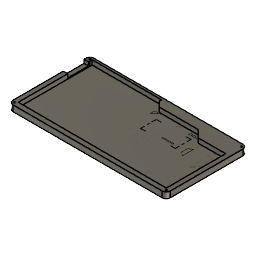
bottom (Autodesk Fusion 360 design; units mm, degrees)
part number: 2026-05-11-22-57-26-323
Autodesk Fusion 360 part; units mm, degrees
sketch "Sketch2" plane through (0, 0, 0) normal (0, 0, 1) x (1, 0, 0)
  line L0 (-104.034, 27.8554) -> (-104.2569, -127.6847)
  line L1 (47.3447, 27.8244) -> (-104.034, 27.8554)
  line L2 (58.096, 16.7354) -> (47.3447, 27.8244)
  line L3 (143.396, 16.6254) -> (58.096, 16.7354)
  line L4 (158.776, 0.9754) -> (143.396, 16.6254)
  line L5 (218.636, 1.1054) -> (158.776, 0.9754)
  line L6 (218.786, -128.4147) -> (218.636, 1.1054)
  line L7 (-104.2569, -127.6847) -> (218.786, -128.4147)
  line L8 (-114.034, 37.8554) -> (228.636, 37.8554)
  line L9 (228.636, 37.8554) -> (228.636, -138.4147)
  line L10 (228.636, -138.4147) -> (-114.034, -138.4147)
  line L11 (-114.034, -138.4147) -> (-114.034, 37.8554)
  circle A0 centre (-108.034, 31.8554) radius 1.75
  circle A1 centre (222.636, 31.8554) radius 1.75
  circle A2 centre (-108.034, -132.4147) radius 1.75
  circle A3 centre (222.636, -132.4147) radius 1.75
  dimension "d24" = 10
  dimension "d25" = 10
  dimension "d26" = 10
  dimension "d27" = 10
  dimension "d32" = 3.5
  dimension "d33" = 6
  dimension "d34" = 6
  dimension "d35" = 6
  dimension "d36" = 6
  dimension "d37" = 3.5
  dimension "d38" = 3.5
  dimension "d39" = 6
  dimension "d40" = 6
  dimension "d41" = 3.5
  dimension "d42" = 6
  dimension "d43" = 6
  constraint horizontal L8
  constraint vertical L9
  constraint horizontal L10
  constraint vertical L11
  measures "d24" vertical distance of L0.start L8.start
  measures "d25" distance of L0.start L11
  measures "d26" horizontal distance of L5.start L8.end
  measures "d27" vertical distance of L6.start L9.end
  measures "d32" diameter of A0
  measures "d33" distance of L8 A0.centre
  measures "d34" distance of L11 A0.centre
  measures "d35" distance of L9 A1.centre
  measures "d36" distance of L8 A1.centre
  measures "d37" diameter of A1
  measures "d38" diameter of A2
  measures "d39" distance of L11 A2.centre
  measures "d40" distance of L10 A2.centre
  measures "d41" diameter of A3
  measures "d42" distance of L9 A3.centre
  measures "d43" distance of L10 A3.centre
extrude "Extrude2" add sketch "Sketch2" along normal blind 3 contours L0 L1 L2 L3 L4 L5 L6 L7
extrude "Extrude3" add sketch "Sketch2" along normal blind 13 contours L8 L9 L10 L11 | A0 | A1 | A2 | A3
sketch "Sketch5" plane through (0, 0, 13) normal (0, 0, 1) x (-1, 0, 0)
  line L0 (-218.786, 128.4147) -> (104.2569, 127.6847)
  line L1 (104.2569, 127.6847) -> (104.034, -27.8554)
  line L2 (104.034, -27.8554) -> (-47.3447, -27.8244)
  line L3 (-47.3447, -27.8244) -> (-58.096, -16.7354)
  line L4 (-58.096, -16.7354) -> (-143.396, -16.6254)
  line L5 (-143.396, -16.6254) -> (-158.776, -0.9754)
  line L6 (-158.776, -0.9754) -> (-218.636, -1.1054)
  line L7 (-218.636, -1.1054) -> (-218.786, 128.4147)
  line L8 (114.034, 138.4147) -> (-228.636, 138.4147)
  line L9 (-228.636, 138.4147) -> (-228.636, -37.8554)
  line L10 (-228.636, -37.8554) -> (114.034, -37.8554)
  line L11 (114.034, -37.8554) -> (114.034, 138.4147)
  circle A0 centre (108.034, -31.8554) radius 1.75
  line L12 (114.034, -37.8554) -> (-228.636, -37.8554)
  line L13 (114.034, 138.4147) -> (114.034, -37.8554)
  circle A1 centre (108.034, 132.4147) radius 1.75
  line L14 (-228.636, 138.4147) -> (114.034, 138.4147)
  circle A2 centre (-222.636, 132.4147) radius 1.75
  line L15 (-228.636, -37.8554) -> (-228.636, 138.4147)
  circle A3 centre (-222.636, -31.8554) radius 1.75
  dimension "d44" = 3.5
  dimension "d45" = 6
  dimension "d46" = 6
  dimension "d47" = 3.5
  dimension "d48" = 6
  dimension "d49" = 6
  dimension "d50" = 3.5
  dimension "d51" = 6
  dimension "d52" = 6
  dimension "d53" = 3.5
  dimension "d54" = 6
  dimension "d55" = 6
  measures "d44" diameter of A0
  measures "d45" distance of A0.centre L12
  measures "d46" distance of A0.centre L13
  measures "d47" diameter of A1
  measures "d48" distance of A1.centre L14
  measures "d49" distance of L13 A1.centre
  measures "d50" diameter of A2
  measures "d51" distance of A2.centre L15
  measures "d52" distance of L14 A2.centre
  measures "d53" diameter of A3
  measures "d54" distance of L15 A3.centre
  measures "d55" distance of L12 A3.centre
extrude "Extrude4" cut sketch "Sketch5" against normal blind 13 contours A0 | A1 | A2 | A3
fillet "Fillet1" radius 9 4 edges at (-114.034, -138.4147, 6.5) (228.636, -138.4147, 6.5) (228.636, 37.8554, 6.5) (-114.034, 37.8554, 6.5)
sketch "Sketch6" plane through (-114.034, 0, 0) normal (-1, 0, 0) x (0, -1, 0)
  line L0 (-28.8554, 13) -> (-28.8554, 0)
  line L1 (-28.8554, 0) -> (129.4147, 0)
  line L2 (129.4147, 0) -> (129.4147, 13)
  line L3 (129.4147, 13) -> (-28.8554, 13)
  line L4 (-25.142, 13) -> (20, 13)
  line L5 (20, 13) -> (20, 5)
  line L6 (20, 5) -> (-25.142, 5)
  line L7 (-25.142, 5) -> (-25.142, 13)
  constraint horizontal L4
  constraint vertical L5
  constraint horizontal L6
  constraint vertical L7
  constraint coincident L3 L4.start
extrude "Extrude5" cut sketch "Sketch6" against normal blind 50 contours L3 L4 L5 L6 L7
extrude "Extrude6" cut 1 faces at (-3.1149, 27.8347, 6.3333) along direction (0.000205, 1, 0) blind 5
sketch "Sketch7" plane through (0, 0, 0) normal (0, 0, -1) x (1, 0, 0)
  arc A0 (-114.034, -28.8554) -> (-105.034, -37.8554) centre (-105.034, -28.8554) ccw
  line L0 (-105.034, -37.8554) -> (219.636, -37.8554)
  arc A1 (219.636, -37.8554) -> (228.636, -28.8554) centre (219.636, -28.8554) ccw
  line L1 (228.636, -28.8554) -> (228.636, 129.4147)
  arc A2 (228.636, 129.4147) -> (219.636, 138.4147) centre (219.636, 129.4147) ccw
  line L2 (219.636, 138.4147) -> (-105.034, 138.4147)
  arc A3 (-105.034, 138.4147) -> (-114.034, 129.4147) centre (-105.034, 129.4147) ccw
  line L3 (-114.034, 129.4147) -> (-114.034, -28.8554)
  circle A4 centre (-108.034, -31.8554) radius 1.75
  circle A5 centre (222.636, -31.8554) radius 1.75
  circle A6 centre (-108.034, 132.4147) radius 1.75
  circle A7 centre (222.636, 132.4147) radius 1.75
  line L4 (208.4356, -14.7511) -> (211.2583, -11.9169)
  line L5 (211.2583, -11.9169) -> (196.2279, 3.0526)
  line L6 (196.2279, 3.0526) -> (193.4053, 0.2185)
  line L7 (193.4053, 0.2185) -> (208.4356, -14.7511)
  line L8 (212.1042, 1.0407) -> (209.9795, 3.1654)
  line L9 (209.9795, 3.1654) -> (193.7795, -13.1004)
  line L10 (193.7795, -13.1004) -> (195.9949, -15.3067)
  line L11 (195.9949, -15.3067) -> (212.1042, 1.0407)
  line L12 (192.7266, 25.5315) -> (207.7266, 10.5315)
  line L13 (210.555, 13.3599) -> (195.555, 28.3599)
  line L14 (207.7266, 10.5315) -> (210.555, 13.3599)
  line L15 (195.555, 28.3599) -> (192.7266, 25.5315)
  line L16 (211.0851, 25.6248) -> (196.0851, 10.6248)
  line L17 (193.2567, 13.4532) -> (208.2567, 28.4532)
  line L18 (196.0851, 10.6248) -> (193.2567, 13.4532)
  line L19 (208.2567, 28.4532) -> (211.0851, 25.6248)
  line L20 (192.8504, 49.7209) -> (207.8115, 34.8203)
  line L21 (207.8115, 34.8203) -> (210.6179, 37.4996)
  line L22 (210.6179, 37.4996) -> (195.6179, 52.4996)
  line L23 (195.6179, 52.4996) -> (192.8504, 49.7209)
  line L24 (150, -15) -> (165, 0)
  line L25 (165, 0) -> (165, 45)
  line L26 (165, 45) -> (50, 45)
  line L27 (50, 45) -> (50, -15)
  line L28 (50, -15) -> (150, -15)
  line L29 (102.4945, -10.0423) -> (87.4945, -10.0423)
  line L30 (87.4945, -10.0423) -> (82.5368, -15)
  line L31 (102.4945, -10.0423) -> (107.4522, -15)
  line L32 (59.741, -15) -> (50, -5.259)
  line L33 (51.9895, 5) -> (48.0056, 5)
  line L34 (48.0056, 5) -> (48.0056, 15)
  line L35 (48.0056, 15) -> (51.9895, 15)
  line L36 (51.9895, 15) -> (51.9895, 5)
  line L37 (52.0057, 20) -> (47.9943, 20)
  line L38 (47.9943, 20) -> (47.9943, 31)
  line L39 (47.9943, 31) -> (52.0057, 31)
  line L40 (52.0057, 31) -> (52.0057, 20)
  line L41 (130, -17.0109) -> (124, -17.0109)
  line L42 (124, -17.0109) -> (124, -13.027)
  line L43 (124, -13.027) -> (130, -13.027)
  line L44 (130, -13.027) -> (130, -17.0109)
  line L45 (150, -12) -> (145, -12)
  line L46 (145, -12) -> (145, -8)
  line L47 (145, -8) -> (150, -8)
  line L48 (150, -8) -> (150, -12)
  line L49 (143, -12) -> (138, -12)
  line L50 (138, -12) -> (138, -8)
  line L51 (138, -8) -> (143, -8)
  line L52 (143, -8) -> (143, -12)
  line L53 (136, -12) -> (131, -12)
  line L54 (131, -12) -> (131, -8)
  line L55 (131, -8) -> (136, -8)
  line L56 (136, -8) -> (136, -12)
  line L57 (165, 40) -> (157, 35)
  line L58 (157, 35) -> (157, 20)
  line L59 (157, 20) -> (165, 15)
  line L60 (145, 43.0006) -> (121, 43.0006)
  line L61 (121, 43.0006) -> (121, 46.9205)
  line L62 (121, 46.9205) -> (145, 46.9205)
  line L63 (145, 46.9205) -> (145, 43.0006)
  line L64 (142.8009, -1.1999) -> (132.8009, -1.1999)
  line L65 (132.8009, -1.1999) -> (132.8009, -0.1999)
  line L66 (132.8009, -0.1999) -> (142.8009, -0.1999)
  line L67 (142.8009, -0.1999) -> (142.8009, 7.8001)
  line L68 (142.8009, 7.8001) -> (143.8009, 7.8001)
  line L69 (143.8009, 7.8001) -> (143.8009, -1.1999)
  line L70 (143.8009, -1.1999) -> (142.8009, -1.1999)
  line L71 (143.8009, 13.8001) -> (143.8009, 18.8001)
  line L72 (143.8009, 18.8001) -> (143.3009, 18.8001)
  line L73 (143.3009, 18.8001) -> (142.8009, 18.8001)
  line L74 (142.8009, 18.8001) -> (142.8009, 13.8001)
  line L75 (142.8009, 13.8001) -> (143.8009, 13.8001)
  line L76 (143.8009, 23.8001) -> (143.8009, 33.8001)
  line L77 (143.8009, 33.8001) -> (132.8009, 33.8001)
  line L78 (132.8009, 33.8001) -> (132.8009, 32.8001)
  line L79 (132.8009, 32.8001) -> (142.8009, 32.8001)
  line L80 (142.8009, 32.8001) -> (142.8009, 23.8001)
  line L81 (142.8009, 23.8001) -> (143.8009, 23.8001)
  line L82 (67.3195, 8.785) -> (67.3195, -1.2)
  line L83 (67.318, 33.785) -> (68.318, 33.785)
  line L84 (67.318, 24.785) -> (67.318, 33.785)
  line L85 (78.318, 33.785) -> (78.318, 32.785)
  line L86 (67.818, 13.785) -> (68.318, 13.785)
  line L87 (78.318, 32.785) -> (68.318, 32.785)
  line L88 (68.318, 32.785) -> (68.318, 24.785)
  line L89 (68.318, 33.785) -> (78.318, 33.785)
  line L90 (68.318, 24.785) -> (67.318, 24.785)
  line L91 (67.318, 13.785) -> (67.818, 13.785)
  line L92 (78.318, -0.215) -> (68.318, -0.215)
  line L93 (68.318, -0.215) -> (68.318, 8.785)
  line L94 (67.3195, -1.2) -> (78.318, -1.2)
  line L95 (68.318, 13.785) -> (68.318, 18.785)
  line L96 (78.318, -1.2) -> (78.318, -0.215)
  line L97 (67.318, 18.785) -> (67.318, 13.785)
  line L98 (68.318, 8.785) -> (67.3195, 8.785)
  line L99 (68.318, 18.785) -> (67.318, 18.785)
  line L100 (150, -16) -> (166, -1)
  line L101 (166, -1) -> (166, 16)
  line L102 (166, 16) -> (166, 46)
  line L103 (166, 46) -> (145, 46)
  line L104 (121, 46) -> (49, 46)
  line L105 (49, 46) -> (49, 31)
  line L106 (49, 20) -> (49, 15)
  line L107 (49, 5) -> (49, -16)
  line L108 (49, -16) -> (81.5, -16)
  line L109 (81.5, -16) -> (82.5368, -15)
  line L110 (107.4522, -15) -> (108.4514, -15.9992)
  line L111 (108.4514, -15.9992) -> (124, -15.9992)
  line L112 (130, -15.9992) -> (150, -16)
  line L113 (132.8009, 28.0219) -> (77.8009, 28.0219)
  line L114 (77.8009, 28.0219) -> (77.8009, 25.9318)
  line L115 (77.8009, 25.9318) -> (132.8009, 25.9318)
  line L116 (132.8009, 25.9318) -> (132.8009, 28.0219)
  line L117 (110.0502, 25.9318) -> (108.5088, 28.0219)
  line L118 (196.1163, 34.666) -> (193.2879, 37.4944)
  line L119 (211.1163, 49.666) -> (196.1163, 34.666)
  line L120 (193.2879, 37.4944) -> (208.2879, 52.4944)
  line L121 (208.2879, 52.4944) -> (211.1163, 49.666)
  dimension "d64" = 4
  dimension "d66" = 4
  dimension "d68" = 4
  dimension "d69" = 4
  constraint perpendicular L4 L5
  constraint perpendicular L5 L6
  constraint perpendicular L6 L7
  constraint perpendicular L7 L9
  constraint perpendicular L9 L10
  constraint perpendicular L13 L14
  constraint perpendicular L13 L15
  constraint perpendicular L12 L15
  constraint perpendicular L17 L18
  constraint perpendicular L17 L19
  constraint perpendicular L16 L19
  constraint perpendicular L20 L23
  constraint vertical L25
  constraint perpendicular L25 L26
  constraint perpendicular L26 L27
  constraint perpendicular L27 L28
  constraint parallel L28 L29
  constraint coincident L28 L30.end
  constraint coincident L28 L31.end
  constraint coincident L28 L32.start
  constraint coincident L27 L32.end
  constraint horizontal L33
  constraint vertical L34
  constraint horizontal L35
  constraint vertical L36
  constraint horizontal L37
  constraint vertical L38
  constraint horizontal L39
  constraint vertical L40
  constraint horizontal L41
  constraint vertical L42
  constraint horizontal L43
  constraint vertical L44
  constraint horizontal L45
  constraint vertical L46
  constraint horizontal L47
  constraint vertical L48
  constraint horizontal L49
  constraint vertical L50
  constraint horizontal L51
  constraint vertical L52
  constraint horizontal L53
  constraint vertical L54
  constraint horizontal L55
  constraint vertical L56
  constraint coincident L25 L57.start
  constraint vertical L58
  constraint coincident L25 L59.end
  constraint horizontal L60
  constraint vertical L61
  constraint horizontal L62
  constraint vertical L63
  constraint horizontal L64
  constraint perpendicular L64 L65
  constraint perpendicular L65 L66
  constraint perpendicular L66 L67
  constraint perpendicular L67 L68
  constraint perpendicular L66 L69
  constraint perpendicular L69 L70
  constraint perpendicular L66 L71
  constraint perpendicular L71 L72
  constraint parallel L66 L73
  constraint perpendicular L73 L74
  constraint perpendicular L74 L75
  constraint perpendicular L73 L76
  constraint perpendicular L76 L77
  constraint perpendicular L73 L78
  constraint perpendicular L76 L79
  constraint perpendicular L79 L80
  constraint perpendicular L76 L81
  constraint perpendicular L85 L89
  constraint perpendicular L85 L87
  constraint perpendicular L87 L88
  constraint perpendicular L88 L90
  constraint perpendicular L84 L87
  constraint perpendicular L83 L84
  constraint perpendicular L87 L97
  constraint perpendicular L91 L97
  constraint parallel L86 L87
  constraint perpendicular L86 L95
  constraint perpendicular L95 L99
  constraint perpendicular L82 L86
  constraint perpendicular L82 L94
  constraint perpendicular L86 L96
  constraint perpendicular L82 L92
  constraint perpendicular L92 L93
  constraint perpendicular L82 L98
  constraint parallel L25 L101
  constraint perpendicular L26 L102
  constraint coincident L63 L103.end
  constraint perpendicular L63 L103
  constraint coincident L61 L104.start
  constraint perpendicular L61 L104
  constraint coincident L39 L105.end
  constraint perpendicular L39 L105
  constraint coincident L37 L106.start
  constraint coincident L35 L106.end
  constraint perpendicular L35 L106
  constraint coincident L33 L107.start
  constraint perpendicular L33 L107
  constraint perpendicular L107 L108
  constraint parallel L31 L110
  constraint coincident L42 L111.end
  constraint perpendicular L42 L111
  constraint coincident L44 L112.start
  constraint perpendicular L113 L114
  constraint perpendicular L115 L116
  constraint coincident L115 L117.start
  constraint coincident L113 L117.end
  constraint perpendicular L118 L120
  constraint perpendicular L120 L121
  constraint perpendicular L119 L121
  measures "d64" distance of L5 L7
  measures "d66" distance of L12 L13
  measures "d68" distance of L16 L17
  measures "d69" distance of L119 L120
extrude "Extrude7" cut sketch "Sketch7" against normal blind 1 contours L4 L5 L7 L11 | L7 L9 L10 L11 | L5 L7 L9 L11 | L5 L8 L9 L11 | L5 L6 L7 L9 | L12 L13 L15 L17 | L12 L13 L16 L17 | L12 L16 L17 L18 | L12 L13 L14 L16 | L13 L16 L17 L19 | L20 L22 L23 L120 | L20 L22 L119 L120 | L20 L118 L119 L120 | L20 L21 L22 L119 | L22 L119 L120 L121 | L24 L25 L26 L28 L44 L63 L100 L101 L102 L103 L112 | L28 L41 L42 L44 | L28 L42 L43 L44 | L28 L42 L110 L111 | L28 L29 L30 L31 | L27 L28 L33 L107 L108 L109 | L26 L60 L61 L63 | L26 L61 L62 L63 | L26 L27 L39 L61 L104 L105 | L27 L33 L34 L35 | L27 L33 L35 L36 | L27 L37 L39 L40 | L27 L37 L38 L39 | L27 L35 L37 L106
extrude "Extrude8" cut sketch "Sketch7" against normal blind 1.5 contours L25 L57 L58 L59 | L27 L28 L32 | L45 L46 L47 L48 | L49 L50 L51 L52 | L53 L54 L55 L56 | L64 L65 L66 L67 L68 L69 L70 | L71 L72 L73 L74 L75 | L76 L77 L78 L79 L80 L81 | L82 L92 L93 L94 L96 L98 | L83 L84 L85 L87 L88 L89 L90 | L86 L91 L95 L97 L99 | L113 L115 L116 L117
extrude "Extrude9" cut sketch "Sketch7" against normal blind 1 contours L113 L114 L115 L117
